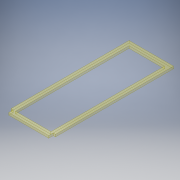
# Autodesk Inventor part: tank_lid_main
Saved by Autodesk Inventor 2018.1 (Build 221171000, 171)
## iProperties
Created: 2017-08-15
Part Number: tank_lid_main
Material: PVC-Piping
Document SubType Name: Modeling
Designer: Tom
Density: 1.4 g/cm^3
Appearance: Clear - Yellow
Mass: 173.578 g
Surface Area: 651.52 cm^2
Volume: 123.984 cm^3
Author: Tom
Autodesk Inventor part; units mm, degrees
ref_plane "YZ Plane" through (0, 0, 0) normal (1, 0, 0) x (0, 1, 0)
ref_plane "XZ Plane" through (0, 0, 0) normal (0, 1, 0) x (-1, 0, 0)
ref_plane "Work Plane1" through (0, 0, 5) normal (0, 0, 1) x (1, 0, 0)
sketch "Sketch2" plane through (0, 0, 5) normal (0, 0, 1) x (1, 0, 0)
  line L0 (5, 278.5) -> (104, 278.5) construction
  line L1 (104, 278.5) -> (104, 5.5) construction
  line L2 (104, 5.5) -> (5, 5.5) construction
  line L3 (5, 5.5) -> (5, 278.5) construction
  line L4 (110, 284) -> (0, 284) projected
  line L5 (0, 0) -> (110, 0) projected
  line L6 (0, 284) -> (0, 0) projected
  line L7 (15, 15.5) -> (94, 15.5)
  line L8 (94, 15.5) -> (94, 268.5)
  line L9 (94, 268.5) -> (15, 268.5)
  line L10 (15, 268.5) -> (15, 15.5)
  line L11 (5, 5.5) -> (10, 5.5) construction
  line L12 (10, 5.5) -> (10, 15.5) construction
  line L13 (104, 5.5) -> (99, 5.5) construction
  line L14 (99, 5.5) -> (99, 15.5) construction
  line L15 (10, 5.5) -> (10, 15.5)
  line L16 (10, 15.5) -> (5, 15.5)
  line L17 (5, 15.5) -> (5, 278.5)
  line L18 (5, 278.5) -> (104, 278.5)
  line L19 (99, 5.5) -> (99, 15.5)
  line L20 (99, 15.5) -> (104, 15.5)
  line L21 (104, 15.5) -> (104, 278.5)
  line L22 (99, 5.5) -> (10, 5.5)
  dimension "d4" = 99
  dimension "d5" = 273
  dimension "d6" = 5.5
  dimension "d7" = 5.5
  dimension "d8" = 5
  dimension "d9" = 79
  dimension "d10" = 253
  dimension "d11" = 10
  dimension "d12" = 10
  dimension "d13" = 5
  dimension "d14" = 10
  dimension "d15" = 5
  dimension "d16" = 10
  constraints: 40 end point, 5 collinear, 5 perpendicular, 4 parallel, 4 point on line, 2 horizontal
  measures "d4" distance of L1.end L2.end
  measures "d5" distance of L0.end L1.end
  measures "d6" distance between parallel lines of L4 L0
  measures "d7" distance between parallel lines of L5 L2
  measures "d8" distance between parallel lines of L6 L3
  measures "d9" distance of L7.start L7.end
  measures "d10" distance of L9.end L7.start
  measures "d11" distance between parallel lines of L2 L7
  measures "d12" distance between parallel lines of L3 L10
  measures "d13" distance of L2.end L11.end
  measures "d14" distance of L11.end L12.end
  measures "d15" distance of L1.end L13.end
  measures "d16" distance of L13.end L14.end
extrude "Extrusion2" add sketch "Sketch2" along normal blind 5
equation "\"d4\" = tankw - 2 * slack"
equation "\"d5\" = -sensorsupportl + tankl - pvct - 2 * slack"
equation "\"d9\" = -2 * slack + tankw - 2 * bracketw"
equation "\"d10\" = -2 * slack - pvct + tankl - sensorsupportl - 2 * bracketw"
equation "\"d11\" = bracketw"
equation "\"d12\" = bracketw"
equation "\"d13\" = pvct"
equation "\"d14\" = bracketw"
equation "\"d15\" = pvct"
equation "\"d16\" = bracketw"
equation "\"d17\" = pvct"
equation "\"lcsd\" = 19.05"
equation "\"lcwd1\" = 25"
equation "\"lcwd2\" = 34"
equation "\"lch1\" = 39"
equation "\"lcwd3\" = 43"
equation "\"dia1\" = 6"
equation "\"td\" = 18"
equation "\"bhh\" = 6"
equation "\"sw\" = 25"
equation "\"sh\" = 31"
equation "\"spacert\" = 2"
equation "\"pvct\" = 5"
equation "\"tankl\" = 379"
equation "\"dia4\" = 11"
equation "\"dia3\" = 8"
equation "\"play\" = 9"
equation "\"holeh\" = 26"
equation "\"slack\" = 0.5"
equation "\"surroundt\" = 5"
equation "\"play2\" = 3"
equation "\"diaair\" = 32"
equation "\"diaph\" = 32"
equation "\"diawater\" = 25"
equation "\"diacucl\" = 32"
equation "\"diahcl\" = 32"
equation "\"diaoverflow\" = 25"
equation "\"diasurroundhole\" = 42"
equation "\"bracketw\" = 10"
equation "\"bracketwbottom\" = 6"
equation "\"diagrate\" = 12"
equation "\"gratespacing\" = 12.02082"
equation "\"bottomdist\" = 9.6355"
equation "\"sidedist\" = 13.9375"
equation "\"nett\" = 1"
equation "\"nethole\" = 16"
equation "\"netside\" = 3.5"
equation "\"nettop\" = 7"
equation "\"netholespacing\" = 2"
equation "\"diaetape\" = 32"
equation "\"tankw\" = 100"
equation "\"sensorsupportl\" = 100"
body "Solid1"
